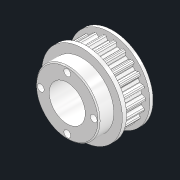
# Autodesk Inventor part: base2
Saved by Autodesk Inventor 2022 (Build 260153000, 153)
## iProperties
Created: 2021-07-14
Part Number: base2
Material: ABS プラスチック
Document SubType Name: Modeling
Designer: yuta0
Density: 1.06 g/cm^3
Appearance: 滑らか - 白
購入先: 印刷
在庫数: 0.0
Author: yuta0
Autodesk Inventor part; units mm, degrees
ref_plane "YZ Plane" through (0, 0, 0) normal (1, 0, 0) x (0, 1, 0)
ref_plane "XZ Plane" through (0, 0, 0) normal (0, 1, 0) x (-1, 0, 0)
ref_plane "XY Plane" through (0, 0, 0) normal (0, 0, 1) x (1, 0, 0)
sketch "スケッチ1" plane through (0, 0, 0) normal (0, 0, 1) x (1, 0, 0)
  circle A0 centre (0, 0) radius 17.507 construction
  circle A1 centre (0, 0) radius 17.025
  circle A2 centre (0, 0) radius 15.255
  line L0 (-1.625, 17.4315) -> (1.625, 17.4315) construction
  line L1 (-24.5099, 0) -> (24.5099, 0) projected
  circle A3 centre (1.625, 17.4315) radius 3.275
  circle A4 centre (-1.625, 17.4315) radius 3.275
  point P0 (0, 17.025)
  point P1 (0.8032, 15.2339)
  point P2 (1.6142, 16.9484)
  point P3 (-1.6142, 16.9484)
  point P4 (-0.8032, 15.2339)
  dimension "d1" = 35.0141
  dimension "d2" = 0.482
  dimension "d3" = 1.77
  dimension "d5" = 6.55
  dimension "d6" = 3.25
  dimension "d7" = 6.55
  constraints: 4 centre point, 3 coincident, 2 end point, 2 point on circle, 1 parallel, 1 vertical alignment, 3 other
  measures "d1" diameter of A0
  measures "d5" diameter of A3
  measures "d6" distance of L0.start L0.end
  measures "d7" diameter of A4
extrude "押し出し1" add sketch "スケッチ1" against normal blind 11 contours L1 A2 A3 A1 | A1 L1 A2 | A3 A2 A4 A1 | A1 A4 A2 L1 | L1 A2 A4 A3 | A2 L1 | A4 A2 A3 A1 | A3 A4 A2 | A1 A3 A2 A4 | A4 A3 A2 | A4 A2 A3
extrude "押し出し2" cut sketch "スケッチ1" against normal through all contours A4 A2 A3 A1 picked at (0.0893, 16.4285)
fillet "フィレット1" radius 0.55 2 edges at (1.6142, 16.9484, -5.5) (-1.6142, 16.9484, -5.5)
fillet "フィレット2" radius 0.25 2 edges at (0.8032, 15.2339, -5.5) (-0.8032, 15.2339, -5.5)
pattern_circular "円形状パターン1" count 22 over 360 about axis through (0, 0, -10) along (0, 0, 1) of "押し出し2", "フィレット1", "フィレット2"
sketch "スケッチ8" plane through (0, 0, -11) normal (0, 0, -1) x (-1, 0, 0)
  circle A0 centre (0, 0) radius 19.025
  arc A1 (6.7855, -15.6144) -> (7.3571, -15.3534) centre (0, 0) ccw projected
  dimension "d66" = 17.025
  dimension "d67" = 38.0501
  constraints: 1 centre point, 1 coincident
  measures "d66" radius of A1
  measures "d67" diameter of A0
extrude "押し出し6" add sketch "スケッチ8" along normal blind 1.5
sketch "スケッチ11" plane through (0, 0, 0) normal (0, 0, 1) x (1, 0, 0)
  circle A0 centre (0, 0) radius 19.025 projected
extrude "押し出し9" add sketch "スケッチ11" along normal blind 2
sketch "スケッチ12" plane through (0, 0, 2) normal (0, 0, 1) x (1, 0, 0)
  circle A0 centre (0, 0) radius 15
  dimension "d70" = 30
  constraints: 1 centre point, 1 coincident
  measures "d70" diameter of A0
extrude "押し出し10" add sketch "スケッチ12" along normal blind 7
sketch "スケッチ2" plane through (0, 0, -12.5) normal (0, 0, -1) x (1, 0, 0)
  circle A0 centre (0, 0) radius 12.5
  point P0 (0, 12.5)
  point P1 (-12.5, 0)
  point P2 (0, -12.5)
  point P3 (12.5, 0)
  dimension "d17" = 25
  dimension "d20" = 360
  constraints: 1 coincident, 1 vertical alignment, 7 other
hole "穴1" at (0, -12.5, -12.5) at (-12.5, 0, -12.5) at (0, 12.5, -12.5) at (12.5, 0, -12.5) direction (0, 0, 1) diameter 3.2 end through all clearance for "Socket Head Cap Screw" size "M3" standard "Ansi Metric M Profile"
chamfer "面取り4" distance 0.5 angle 45 1 edges at (-15, 0, 9)
sketch "スケッチ13" plane through (0, 0, 9) normal (0, 0, 1) x (1, 0, 0)
  circle A0 centre (0, 0) radius 8.5
  dimension "d76" = 17
  constraints: 1 centre point, 1 coincident
  measures "d76" diameter of A0
extrude "押し出し11" cut sketch "スケッチ13" against normal through all
equation "\"d7\" = d5"
